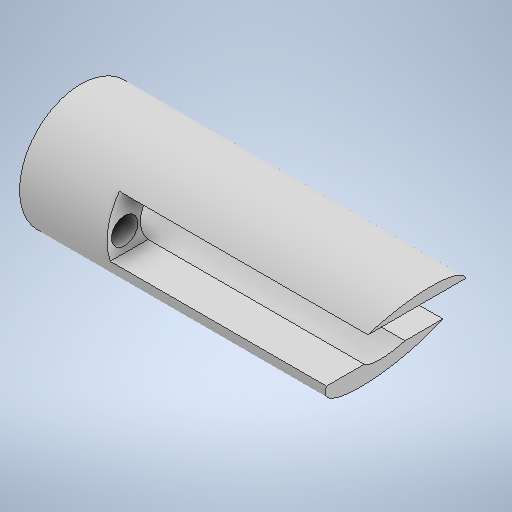
# Autodesk Inventor part: Main_tip_coupler
Saved by Autodesk Inventor 2026.2 (Build 302298010, 298A)
## iProperties
Created: 2026-05-11
Part Number: Main_tip_coupler
Material: Generic
Document SubType Name: Modeling
Designer: piete
Density: 1 g/cm^3
Appearance: Default
Author: piete
Autodesk Inventor part; units mm, degrees
ref_plane "YZ Plane" through (0, 0, 0) normal (1, 0, 0) x (0, 1, 0)
ref_plane "XZ Plane" through (0, 0, 0) normal (0, 1, 0) x (-1, 0, 0)
ref_plane "XY Plane" through (0, 0, 0) normal (0, 0, 1) x (1, 0, 0)
sketch "Sketch1" plane through (0, 0, 0) normal (1, 0, 0) x (0, 1, 0)
  circle A0 centre (0, 0) radius 3.5
  dimension "d0" = 7
  constraints: 1 centre point, 1 coincident
  measures "d0" diameter of A0
extrude "Extrusion1" add sketch "Sketch1" along normal blind 20
sketch "Sketch2" plane through (20, 0, 0) normal (1, 0, 0) x (0, 0, -1)
  line L0 (-3.5, 2.1) -> (3.5, 2.1)
  line L1 (3.5, 2.1) -> (3.5, -1.1)
  line L2 (3.5, -1.1) -> (-3.5, -1.1)
  line L3 (-3.5, -1.1) -> (-3.5, 2.1)
  point P0 (0, 0)
  dimension "d3" = 7
  dimension "d4" = 3.2
  dimension "d5" = 2.1
  dimension "d6" = 3.5
  constraints: 8 end point, 2 parallel, 1 horizontal, 1 perpendicular
  measures "d3" distance of L1.end L2.end
  measures "d4" distance of L0.end L1.end
  measures "d5" distance from line of point (0, 0) L0
  measures "d6" distance from line of point (0, 0) L1
extrude "Extrusion2" cut sketch "Sketch2" against normal blind 15
sketch "Sketch3" plane through (0, 0, 0) normal (-1, 0, 0) x (0, 0, 1)
  circle A0 centre (0, 0) radius 1.6
  dimension "d9" = 3.2
  constraints: 1 centre point, 1 coincident
  measures "d9" diameter of A0
extrude "Extrusion3" cut sketch "Sketch3" against normal through all
sketch "Sketch4" plane through (0, 0, 0) normal (0, 0, 1) x (1, 0, 0)
  line L0 (20, 2.1) -> (20, 3.5) projected
  line L1 (20, 3.5) -> (15.9585, -3.5)
  line L2 (0, -3.5) -> (20, -3.5) projected
  line L3 (20, 3.5) -> (28.0829, 3.5) construction
  line L4 (15.9585, -3.5) -> (20, -3.5)
  line L5 (20, 3.5) -> (20, -3.5)
  point P0 (0, 0)
  dimension "d12" = 120
  constraints: 8 end point, 2 point on line, 1 equal length, 1 horizontal, 1 perpendicular
  measures "d12" angle of L1 L3
extrude "Extrusion4" cut sketch "Sketch4" along normal through all both and the other way through all
sketch "Sketch5" plane through (0, 0, 0) normal (-1, 0, 0) x (0, 0, 1)
  circle A0 centre (2.5, 0) radius 0.75
  circle A1 centre (-2.5, 0) radius 0.75
  circle A2 centre (0, 0) radius 3.5 projected
  dimension "d15" = 1.5
  dimension "d16" = 1.5
  dimension "d17" = 2.5
  dimension "d18" = 2.5
  dimension "d19" = 0
  dimension "d20" = 0
  constraints: 2 centre point
  measures "d15" diameter of A0
  measures "d16" diameter of A1
  measures "d17" distance of A2.centre A1.centre
  measures "d18" distance of point (0, 0) A0.centre
  measures "d19" vertical distance of A1.centre A0.centre
  measures "d20" vertical distance of point (0, 0) A1.centre
extrude "Extrusion5" cut sketch "Sketch5" against normal through all contours A0 | A1
equation "\"d6\" = 0.5 * d3"
body "Solid1"
